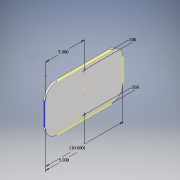
# Autodesk Inventor part: Frame
Saved by Autodesk Inventor 2018.2 (Build 222227000, 227)
## iProperties
Created: 2018-02-01
Part Number: Frame
Material: ABS Plastic
Document SubType Name: Modeling
Designer: MIABo
Density: 1.06 g/cm^3
Appearance: Smooth - White
Mass: 511.869 g
Surface Area: 864.604 cm^2
Volume: 482.895 cm^3
Author: MIABo
Autodesk Inventor part; units mm, degrees
ref_plane "YZ Plane" through (0, 0, 0) normal (1, 0, 0) x (0, 1, 0)
ref_plane "XZ Plane" through (0, 0, 0) normal (0, 1, 0) x (-1, 0, 0)
ref_plane "XY Plane" through (0, 0, 0) normal (0, 0, 1) x (1, 0, 0)
sketch "Sketch1" plane through (0, 0, 0) normal (1, 0, 0) x (0, 1, 0)
  line L0 (65.5874, 89.9095) -> (65.5874, -87.8905)
  line L1 (27.4874, -125.9905) -> (-48.7126, -125.9905)
  line L2 (-86.8126, -87.8905) -> (-86.8126, 89.9095)
  line L3 (-48.7126, 128.0095) -> (27.4874, 128.0095)
  arc A0 (27.4874, -125.9905) -> (65.5874, -87.8905) centre (27.4874, -87.8905) ccw
  arc A1 (-86.8126, -87.8905) -> (-48.7126, -125.9905) centre (-48.7126, -87.8905) ccw
  arc A2 (-48.7126, 128.0095) -> (-86.8126, 89.9095) centre (-48.7126, 89.9095) ccw
  arc A3 (65.5874, 89.9095) -> (27.4874, 128.0095) centre (27.4874, 89.9095) ccw
  point P0 (0, 0)
  point P1 (65.5874, 128.0095)
  point P2 (65.5874, -125.9905)
  point P3 (-86.8126, 128.0095)
  dimension "d0" = 254
  dimension "d1" = 152.4
  dimension "d3" = 38.1
  dimension "d36" = 38.1
  dimension "d37" = 38.1
  dimension "d38" = 177.8
  constraints: 8 end point, 8 point on circle, 8 tangent, 6 point on line, 4 centre point, 3 perpendicular, 1 vertical
  measures "d0" distance of point (65.587, 128.009) point (65.587, -125.991)
  measures "d1" distance of point (-86.813, 128.009) point (65.587, 128.009)
  measures "d3" radius of A1
  measures "d36" radius of A2
  measures "d37" radius of A3
  measures "d38" distance of L2.start L2.end
extrude "Extrusion1" add sketch "Sketch1" along normal blind 6.35
sketch "Sketch3" plane through (6.35, 0, 0) normal (1, 0, 0) x (0, 0, -1)
  line L0 (125.9905, -48.7126) -> (125.9905, 27.4874) projected
  line L1 (-128.0095, 27.4874) -> (-128.0095, -48.7126) projected
  line L2 (-89.9095, -86.8126) -> (87.8905, -86.8126) projected
  line L3 (-89.9095, 65.5874) -> (87.8905, 65.5874) projected
  point P0 (0, 0)
  point P1 (-1.0095, -74.1126)
  point P2 (-128.0095, 100.5124)
  point P3 (-128.0095, -51.8876)
  point P4 (87.8905, -86.8126)
  point P5 (-1.0095, 52.8874)
  point P6 (-1.0095, 52.8874)
  point P7 (87.8905, 65.5874)
  dimension "d16" = 254
  dimension "d17" = 127
  dimension "d18" = 12.7
  dimension "d26" = 12.7
  dimension "d27" = 127
  constraints: 1 coincident, 2 other
  measures "d16" distance between parallel lines of L0 L1
  measures "d17" distance from line of L1 point (-1.009, -74.113)
  measures "d27" distance from line of L1 point (-1.009, 52.887)
hole "Hole2" at (6.35, -74.1126, 1.0095) direction (-1, 0, 0) diameter 6.35 end through all
hole "Hole3" at (6.35, 52.8874, 1.0095) direction (-1, 0, 0) diameter 6.35 end through all
body "Solid1"
